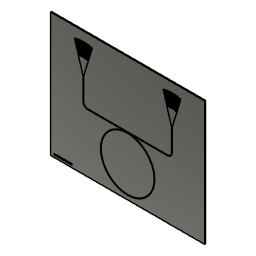
SimpleRes (Autodesk Fusion 360 design; units mm, degrees)
Autodesk Fusion 360 part; units mm, degrees
note: some values were not read from the file. Chosen so that the rebuilt part matches the saved one: which bodies a step acts on.
sketch "Sketch1" plane through (0, 0, 0) normal (0, 1, 0) x (1, 0, 0)
  circle A0 centre (0, 0) radius 30
  circle A1 centre (0, 0) radius 30.5
  line L0 (-45, -30.95) -> (45, -30.95)
  line L1 (-50, -35.95) -> (-50, -60.95)
  line L2 (50, -35.95) -> (50, -60.95)
  arc A2 (-45, -30.95) -> (-50, -35.95) centre (-45, -35.95) ccw
  arc A3 (50, -35.95) -> (45, -30.95) centre (45, -35.95) ccw
  line L3 (49.75, -35.95) -> (49.75, -60.95)
  arc A4 (49.75, -35.95) -> (45, -31.2) centre (45, -35.95) ccw
  line L4 (-45, -31.2) -> (45, -31.2)
  arc A5 (-45, -31.2) -> (-49.75, -35.95) centre (-45, -35.95) ccw
  line L5 (-49.75, -35.95) -> (-49.75, -60.95)
  line L6 (50.25, -35.95) -> (50.25, -60.95)
  arc A6 (50.25, -35.95) -> (45, -30.7) centre (45, -35.95) ccw
  line L7 (-45, -30.7) -> (45, -30.7)
  arc A7 (-45, -30.7) -> (-50.25, -35.95) centre (-45, -35.95) ccw
  line L8 (-50.25, -35.95) -> (-50.25, -60.95)
  line L9 (49.75, -60.95) -> (50.25, -60.95)
  line L10 (50.25, -60.95) -> (60.0334, -92.95)
  line L11 (49.75, -60.95) -> (39.9666, -92.95)
  arc A8 (39.9666, -92.95) -> (60.0334, -92.95) centre (50, -60.95) ccw
  line L12 (-50.25, -60.95) -> (-49.75, -60.95)
  line L13 (-49.75, -60.95) -> (-39.9666, -92.95)
  line L14 (-50.25, -60.95) -> (-60.0334, -92.95)
  arc A9 (-60.0334, -92.95) -> (-39.9666, -92.95) centre (-50, -60.95) ccw
  arc A10 (-55.6371, -78.5703) -> (-44.3629, -78.5703) centre (-50, -60.95) ccw
  arc A11 (-55.698, -78.7608) -> (-44.302, -78.7608) centre (-50, -60.95) ccw
  arc A12 (-55.7589, -78.9512) -> (-44.2411, -78.9512) centre (-50, -60.95) ccw
  arc A13 (-55.8199, -79.1417) -> (-44.1801, -79.1417) centre (-50, -60.95) ccw
  arc A14 (-55.9722, -79.618) -> (-44.0278, -79.618) centre (-50, -60.95) ccw
  arc A15 (-56.0332, -79.8084) -> (-43.9668, -79.8084) centre (-50, -60.95) ccw
  arc A16 (-56.0941, -79.9989) -> (-43.9059, -79.9989) centre (-50, -60.95) ccw
  arc A17 (-56.1551, -80.1894) -> (-43.8449, -80.1894) centre (-50, -60.95) ccw
  arc A18 (-56.3074, -80.6656) -> (-43.6926, -80.6656) centre (-50, -60.95) ccw
  arc A19 (-56.3683, -80.8561) -> (-43.6317, -80.8561) centre (-50, -60.95) ccw
  arc A20 (-56.4293, -81.0466) -> (-43.5707, -81.0466) centre (-50, -60.95) ccw
  arc A21 (-56.4902, -81.2371) -> (-43.5098, -81.2371) centre (-50, -60.95) ccw
  arc A22 (-56.6426, -81.7133) -> (-43.3574, -81.7133) centre (-50, -60.95) ccw
  arc A23 (-56.7035, -81.9038) -> (-43.2965, -81.9038) centre (-50, -60.95) ccw
  arc A24 (-56.7645, -82.0943) -> (-43.2355, -82.0943) centre (-50, -60.95) ccw
  arc A25 (-56.8254, -82.2848) -> (-43.1746, -82.2848) centre (-50, -60.95) ccw
  arc A26 (-56.9778, -82.761) -> (-43.0222, -82.761) centre (-50, -60.95) ccw
  arc A27 (-57.0387, -82.9515) -> (-42.9613, -82.9515) centre (-50, -60.95) ccw
  arc A28 (-57.0996, -83.142) -> (-42.9004, -83.142) centre (-50, -60.95) ccw
  arc A29 (-57.1606, -83.3325) -> (-42.8394, -83.3325) centre (-50, -60.95) ccw
  arc A30 (-57.3129, -83.8087) -> (-42.6871, -83.8087) centre (-50, -60.95) ccw
  arc A31 (-57.3739, -83.9992) -> (-42.6261, -83.9992) centre (-50, -60.95) ccw
  arc A32 (-57.4348, -84.1897) -> (-42.5652, -84.1897) centre (-50, -60.95) ccw
  arc A33 (-57.4958, -84.3802) -> (-42.5042, -84.3802) centre (-50, -60.95) ccw
  arc A34 (-57.6481, -84.8564) -> (-42.3519, -84.8564) centre (-50, -60.95) ccw
  arc A35 (-57.7091, -85.0469) -> (-42.2909, -85.0469) centre (-50, -60.95) ccw
  arc A36 (-57.77, -85.2374) -> (-42.23, -85.2374) centre (-50, -60.95) ccw
  arc A37 (-57.8309, -85.4279) -> (-42.1691, -85.4279) centre (-50, -60.95) ccw
  arc A38 (-57.9833, -85.9041) -> (-42.0167, -85.9041) centre (-50, -60.95) ccw
  arc A39 (-58.0442, -86.0946) -> (-41.9558, -86.0946) centre (-50, -60.95) ccw
  arc A40 (-58.1052, -86.2851) -> (-41.8948, -86.2851) centre (-50, -60.95) ccw
  arc A41 (-58.1661, -86.4756) -> (-41.8339, -86.4756) centre (-50, -60.95) ccw
  arc A42 (-58.3185, -86.9518) -> (-41.6815, -86.9518) centre (-50, -60.95) ccw
  arc A43 (-58.3794, -87.1423) -> (-41.6206, -87.1423) centre (-50, -60.95) ccw
  arc A44 (-58.4403, -87.3328) -> (-41.5597, -87.3328) centre (-50, -60.95) ccw
  arc A45 (-58.5013, -87.5233) -> (-41.4987, -87.5233) centre (-50, -60.95) ccw
  arc A46 (-58.6536, -87.9995) -> (-41.3464, -87.9995) centre (-50, -60.95) ccw
  arc A47 (-58.7146, -88.19) -> (-41.2854, -88.19) centre (-50, -60.95) ccw
  arc A48 (-58.7755, -88.3805) -> (-41.2245, -88.3805) centre (-50, -60.95) ccw
  arc A49 (-58.8365, -88.571) -> (-41.1635, -88.571) centre (-50, -60.95) ccw
  arc A50 (-58.9888, -89.0472) -> (-41.0112, -89.0472) centre (-50, -60.95) ccw
  arc A51 (-59.0498, -89.2377) -> (-40.9502, -89.2377) centre (-50, -60.95) ccw
  arc A52 (-59.1107, -89.4282) -> (-40.8893, -89.4282) centre (-50, -60.95) ccw
  arc A53 (-59.1716, -89.6186) -> (-40.8284, -89.6186) centre (-50, -60.95) ccw
  arc A54 (-59.324, -90.0949) -> (-40.676, -90.0949) centre (-50, -60.95) ccw
  arc A55 (-59.3849, -90.2854) -> (-40.6151, -90.2854) centre (-50, -60.95) ccw
  arc A56 (-59.4459, -90.4758) -> (-40.5541, -90.4758) centre (-50, -60.95) ccw
  arc A57 (-59.5068, -90.6663) -> (-40.4932, -90.6663) centre (-50, -60.95) ccw
  arc A58 (-59.6592, -91.1426) -> (-40.3408, -91.1426) centre (-50, -60.95) ccw
  arc A59 (-59.7201, -91.333) -> (-40.2799, -91.333) centre (-50, -60.95) ccw
  arc A60 (-59.7811, -91.5235) -> (-40.2189, -91.5235) centre (-50, -60.95) ccw
  arc A61 (-59.842, -91.714) -> (-40.158, -91.714) centre (-50, -60.95) ccw
  arc A62 (-59.9943, -92.1902) -> (-40.0057, -92.1902) centre (-50, -60.95) ccw
  arc A63 (-60.0553, -92.3807) -> (-39.9447, -92.3807) centre (-50, -60.95) ccw
  arc A64 (-60.1162, -92.5712) -> (-39.8838, -92.5712) centre (-50, -60.95) ccw
  arc A65 (-60.1772, -92.7617) -> (-39.8228, -92.7617) centre (-50, -60.95) ccw
  arc A66 (44.3629, -78.5703) -> (55.6371, -78.5703) centre (50, -60.95) ccw
  arc A67 (44.302, -78.7608) -> (55.698, -78.7608) centre (50, -60.95) ccw
  arc A68 (44.2411, -78.9512) -> (55.7589, -78.9512) centre (50, -60.95) ccw
  arc A69 (44.1801, -79.1417) -> (55.8199, -79.1417) centre (50, -60.95) ccw
  arc A70 (44.0278, -79.618) -> (55.9722, -79.618) centre (50, -60.95) ccw
  arc A71 (43.9668, -79.8084) -> (56.0332, -79.8084) centre (50, -60.95) ccw
  arc A72 (43.9059, -79.9989) -> (56.0941, -79.9989) centre (50, -60.95) ccw
  arc A73 (43.8449, -80.1894) -> (56.1551, -80.1894) centre (50, -60.95) ccw
  arc A74 (43.6926, -80.6656) -> (56.3074, -80.6656) centre (50, -60.95) ccw
  arc A75 (43.6317, -80.8561) -> (56.3683, -80.8561) centre (50, -60.95) ccw
  arc A76 (43.5707, -81.0466) -> (56.4293, -81.0466) centre (50, -60.95) ccw
  arc A77 (43.5098, -81.2371) -> (56.4902, -81.2371) centre (50, -60.95) ccw
  arc A78 (43.3574, -81.7133) -> (56.6426, -81.7133) centre (50, -60.95) ccw
  arc A79 (43.2965, -81.9038) -> (56.7035, -81.9038) centre (50, -60.95) ccw
  arc A80 (43.2355, -82.0943) -> (56.7645, -82.0943) centre (50, -60.95) ccw
  arc A81 (43.1746, -82.2848) -> (56.8254, -82.2848) centre (50, -60.95) ccw
  arc A82 (43.0222, -82.761) -> (56.9778, -82.761) centre (50, -60.95) ccw
  arc A83 (42.9613, -82.9515) -> (57.0387, -82.9515) centre (50, -60.95) ccw
  arc A84 (42.9004, -83.142) -> (57.0996, -83.142) centre (50, -60.95) ccw
  arc A85 (42.8394, -83.3325) -> (57.1606, -83.3325) centre (50, -60.95) ccw
  arc A86 (42.6871, -83.8087) -> (57.3129, -83.8087) centre (50, -60.95) ccw
  arc A87 (42.6261, -83.9992) -> (57.3739, -83.9992) centre (50, -60.95) ccw
  arc A88 (42.5652, -84.1897) -> (57.4348, -84.1897) centre (50, -60.95) ccw
  arc A89 (42.5042, -84.3802) -> (57.4958, -84.3802) centre (50, -60.95) ccw
  arc A90 (42.3519, -84.8564) -> (57.6481, -84.8564) centre (50, -60.95) ccw
  arc A91 (42.2909, -85.0469) -> (57.7091, -85.0469) centre (50, -60.95) ccw
  arc A92 (42.23, -85.2374) -> (57.77, -85.2374) centre (50, -60.95) ccw
  arc A93 (42.1691, -85.4279) -> (57.8309, -85.4279) centre (50, -60.95) ccw
  arc A94 (42.0167, -85.9041) -> (57.9833, -85.9041) centre (50, -60.95) ccw
  arc A95 (41.9558, -86.0946) -> (58.0442, -86.0946) centre (50, -60.95) ccw
  arc A96 (41.8948, -86.2851) -> (58.1052, -86.2851) centre (50, -60.95) ccw
  arc A97 (41.8339, -86.4756) -> (58.1661, -86.4756) centre (50, -60.95) ccw
  arc A98 (41.6815, -86.9518) -> (58.3185, -86.9518) centre (50, -60.95) ccw
  arc A99 (41.6206, -87.1423) -> (58.3794, -87.1423) centre (50, -60.95) ccw
  arc A100 (41.5597, -87.3328) -> (58.4403, -87.3328) centre (50, -60.95) ccw
  arc A101 (41.4987, -87.5233) -> (58.5013, -87.5233) centre (50, -60.95) ccw
  arc A102 (41.3464, -87.9995) -> (58.6536, -87.9995) centre (50, -60.95) ccw
  arc A103 (41.2854, -88.19) -> (58.7146, -88.19) centre (50, -60.95) ccw
  arc A104 (41.2245, -88.3805) -> (58.7755, -88.3805) centre (50, -60.95) ccw
  arc A105 (41.1635, -88.571) -> (58.8365, -88.571) centre (50, -60.95) ccw
  arc A106 (41.0112, -89.0472) -> (58.9888, -89.0472) centre (50, -60.95) ccw
  arc A107 (40.9502, -89.2377) -> (59.0498, -89.2377) centre (50, -60.95) ccw
  arc A108 (40.8893, -89.4282) -> (59.1107, -89.4282) centre (50, -60.95) ccw
  arc A109 (40.8284, -89.6186) -> (59.1716, -89.6186) centre (50, -60.95) ccw
  arc A110 (40.676, -90.0949) -> (59.324, -90.0949) centre (50, -60.95) ccw
  arc A111 (40.6151, -90.2854) -> (59.3849, -90.2854) centre (50, -60.95) ccw
  arc A112 (40.5541, -90.4758) -> (59.4459, -90.4758) centre (50, -60.95) ccw
  arc A113 (40.4932, -90.6663) -> (59.5068, -90.6663) centre (50, -60.95) ccw
  arc A114 (40.3408, -91.1426) -> (59.6592, -91.1426) centre (50, -60.95) ccw
  arc A115 (40.2799, -91.333) -> (59.7201, -91.333) centre (50, -60.95) ccw
  arc A116 (40.2189, -91.5235) -> (59.7811, -91.5235) centre (50, -60.95) ccw
  arc A117 (40.158, -91.714) -> (59.842, -91.714) centre (50, -60.95) ccw
  arc A118 (40.0057, -92.1902) -> (59.9943, -92.1902) centre (50, -60.95) ccw
  arc A119 (39.9447, -92.3807) -> (60.0553, -92.3807) centre (50, -60.95) ccw
  arc A120 (39.8838, -92.5712) -> (60.1162, -92.5712) centre (50, -60.95) ccw
  arc A121 (39.8228, -92.7617) -> (60.1772, -92.7617) centre (50, -60.95) ccw
  line L15 (-83.2157, 31.3606) -> (-62.7231, 31.3606)
  line L16 (-62.7231, 31.3606) -> (-62.7231, 32.5289)
  line L17 (-62.7231, 32.5289) -> (-83.2157, 32.5289)
  line L18 (-83.2157, 32.5289) -> (-83.2157, 31.3606)
  line L19 (-62.9231, 32.3289) -> (-83.0157, 32.3289)
  line L20 (-83.0157, 32.3289) -> (-83.0157, 31.5606)
  line L21 (-83.0157, 31.5606) -> (-62.9231, 31.5606)
  line L22 (-62.9231, 31.5606) -> (-62.9231, 32.3289)
  line L23 (-73.012, 31.5606) -> (-73.012, 32.3289)
  line L24 (-73.012, 31.5606) -> (-62.9231, 31.5606)
  line L25 (-62.9231, 31.5606) -> (-62.9231, 32.3289)
  line L26 (-62.9231, 32.3289) -> (-73.012, 32.3289)
  line L27 (-73.012, 32.3289) -> (-73.012, 31.5606)
  line L28 (-87.1137, -104.9748) -> (86.8892, -104.9748)
  line L29 (86.8892, -104.9748) -> (86.8892, 35.3192)
  line L30 (86.8892, 35.3192) -> (-87.1137, 35.3192)
  line L31 (-87.1137, 35.3192) -> (-87.1137, -104.9748)
  point P0 (-50, -30.95)
  point P1 (50, -30.95)
  dimension "d1" = 60
  dimension "d2" = 0.5
  dimension "d3" = 30.95
  dimension "d4" = 50
  dimension "d5" = 50
  dimension "d6" = 30
  dimension "d7" = 30
  dimension "d8" = 5
  dimension "d9" = 0.25
  dimension "d10" = -0.25
  dimension "d12" = 107
  dimension "d13" = 107
  dimension "d14" = 32
  dimension "d15" = 32
  dimension "d16" = 107
  dimension "d17" = 107
  dimension "d18" = 32
  dimension "d19" = 32
  dimension "d20" = 18.5
  dimension "d21" = 0.2
  dimension "d22" = 0.4
  dimension "d23" = 0.6
  dimension "d24" = 1.1
  dimension "d25" = 1.3
  dimension "d26" = 1.5
  dimension "d27" = 1.7
  dimension "d28" = 2.2
  dimension "d29" = 2.4
  dimension "d30" = 2.6
  dimension "d31" = 2.8
  dimension "d32" = 3.3
  dimension "d33" = 3.5
  dimension "d34" = 3.7
  dimension "d35" = 3.9
  dimension "d36" = 4.4
  dimension "d37" = 4.6
  dimension "d38" = 4.8
  dimension "d39" = 5
  dimension "d40" = 5.5
  dimension "d41" = 5.7
  dimension "d42" = 5.9
  dimension "d43" = 6.1
  dimension "d44" = 6.6
  dimension "d45" = 6.8
  dimension "d46" = 7
  dimension "d47" = 7.2
  dimension "d48" = 7.7
  dimension "d49" = 7.9
  dimension "d50" = 8.1
  dimension "d51" = 8.3
  dimension "d52" = 8.8
  dimension "d53" = 9
  dimension "d54" = 9.2
  dimension "d55" = 9.4
  dimension "d56" = 9.9
  dimension "d57" = 10.1
  dimension "d58" = 10.3
  dimension "d59" = 10.5
  dimension "d60" = 11
  dimension "d61" = 11.2
  dimension "d62" = 11.4
  dimension "d63" = 11.6
  dimension "d64" = 12.1
  dimension "d65" = 12.3
  dimension "d66" = 12.5
  dimension "d67" = 12.7
  dimension "d68" = 13.2
  dimension "d69" = 13.4
  dimension "d70" = 13.6
  dimension "d71" = 13.8
  dimension "d72" = 14.3
  dimension "d73" = 14.5
  dimension "d74" = 14.7
  dimension "d75" = 14.9
  dimension "d78" = 100
  dimension "d79" = 0
  dimension "d80" = -0.2
  constraint coincident A0.centre A1.centre
  constraint horizontal L0
  constraint perpendicular L0 L1
  constraint perpendicular L0 L2
  constraint coincident P0 L0
  constraint coincident P0 L1
  constraint tangent L0 A2
  constraint tangent L1 A2
  constraint coincident P1 L0
  constraint coincident P1 L2
  constraint tangent L0 A3
  constraint tangent L2 A3
  constraint equal A2 A3
  constraint perpendicular L3 L9
  constraint coincident L2.end A8.centre
  constraint perpendicular L5 L12
  constraint coincident L1.end A9.centre
  constraint coincident L14 A10.start
  constraint coincident L13 A10.end
  constraint horizontal L15
  constraint vertical L16
  constraint horizontal L17
  constraint vertical L18
  constraint coincident L21 L23.start
  constraint coincident L19 L23.end
  constraint perpendicular L19 L23
  constraint horizontal L24
  constraint vertical L25
  constraint horizontal L26
  constraint vertical L27
  constraint horizontal L28
  constraint vertical L29
  constraint horizontal L30
  constraint vertical L31
  measures "d1" diameter of A0
  measures "d3" distance of A0.centre L0
  measures "d4" horizontal distance of A0.centre P1
  measures "d5" horizontal distance of A0.centre P0
  measures "d6" distance of P0 L1.end
  measures "d7" distance of P1 L2.end
  measures "d8" radius of A2
  measures "d12" angle of L9 L10
  measures "d13" angle of L9 L11
  measures "d14" vertical distance of L6.end L10.end
  measures "d15" vertical distance of L2.end L11.end
  measures "d16" angle of L12 L14
  measures "d17" angle of L12 L13
  measures "d18" vertical distance of L5.end L13.end
  measures "d19" vertical distance of L8.end L14.end
  measures "d20" radius of A10
extrude "Extrude1" add sketch "Sketch1" against normal blind 0.22 contours A1 | L0 L1 L2 A2 A3 L6 A6 L7 A7 L8 L9 L12 | L0 L1 L2 A2 A3 L3 A4 L4 A5 L5 L9 L12 | L12 L13 L14 A10 | L9 L10 L11 A66 | L13 L14 A11 A12 | L10 L11 A67 A68 | L13 L14 A13 A14 | L10 L11 A69 A70 | L13 L14 A15 A16 | L10 L11 A71 A72 | L13 L14 A17 A18 | L10 L11 A73 A74 | L13 L14 A19 A20 | L10 L11 A75 A76 | L13 L14 A21 A22 | L10 L11 A77 A78 | L13 L14 A23 A24 | L10 L11 A79 A80 | L13 L14 A25 A26 | L10 L11 A81 A82 | L13 L14 A27 A28 | L10 L11 A83 A84 | L13 L14 A29 A30 | L10 L11 A85 A86 | L13 L14 A31 A32 | L10 L11 A87 A88 | L13 L14 A33 A34 | L10 L11 A89 A90 | L13 L14 A35 A36 | L10 L11 A91 A92 | L13 L14 A37 A38 | L10 L11 A93 A94 | L13 L14 A39 A40 | L10 L11 A95 A96 | L13 L14 A41 A42 | L10 L11 A97 A98 | L13 L14 A43 A44 | L10 L11 A99 A100 | L13 L14 A45 A46 | L10 L11 A101 A102 | L13 L14 A47 A48 | L10 L11 A103 A104 | L13 L14 A49 A50 | L10 L11 A105 A106 | L13 L14 A51 A52 | L10 L11 A107 A108 | L13 L14 A53 A54 | L10 L11 A109 A110 | L13 L14 A55 A56 | L10 L11 A111 A112 | L13 L14 A57 A58 | L10 L11 A113 A114 | L13 L14 A59 A60 | L10 L11 A115 A116 | L13 L14 A61 A62 | L10 L11 A117 A118 | L13 L14 A63 A64 | L10 L11 A119 A120 | L13 L14 A9 A65 | L10 L11 A8 A121 | L15 L16 L17 L18 | L19 L20 L21 L23 L27 makes body 1 at (50.6544, 0, 93.523) makes body 2 at (43.2646, 0, 90.5771) makes body 3 at (56.2613, 0, 88.4323) makes body 4 at (44.2129, 0, 86.2875) makes body 5 at (53.3263, -0.1467, 84.0113) makes body 6 at (47.8373, -0.1467, 81.9389) makes body 7 at (45.749, -0.1467, 79.3657) makes body 8 at (-58.3639, -0.0733, 91.9412) makes body 9 at (-56.6256, -0.1467, 90.1067) makes body 10 at (-56.1507, -0.1467, 87.9585) makes body 11 at (-52.5972, -0.1467, 86.3174) makes body 12 at (-55.2009, -0.1467, 83.6621) makes body 13 at (-52.1627, -0.1467, 81.9389) makes body 14 at (-51.9455, -0.1467, 79.7496) makes body 15 at (-79.8145, 0, -32.0728) makes body 16 at (-45.6353, 0, 79.8529) makes body 17 at (-45.1612, 0, 81.9978) makes body 18 at (-55.313, 0, 84.1426) makes body 19 at (-55.7871, 0, 86.2875) makes body 20 at (-56.2613, 0, 88.4323) makes body 21 at (-56.7354, 0, 90.5771) makes body 22 at (-49.3456, 0, 93.523) makes body 23 at (54.3647, 0, 79.8529) makes body 24 at (45.1612, 0, 81.9978) makes body 25 at (55.313, 0, 84.1426) makes body 26 at (43.0349, -0.0733, 86.6219) makes body 27 at (43.6118, -0.1467, 89.0326) makes body 28 at (46.8597, -0.1467, 91.7905) makes body 29 at (46.6425, -0.1467, 93.9798) makes body 30 at (41.6361, -0.0733, 91.9412) makes body 31 at (43.3744, -0.1467, 90.1067) makes body 32 at (43.8493, -0.1467, 87.9585) makes body 33 at (53.63, -0.1467, 86.1903) makes body 34 at (55.0759, 0, 83.0702) makes body 35 at (45.3982, 0, 80.9254) makes body 36 at (-58.7291, -0.0733, 93.3301) makes body 37 at (-49.3673, 0, 92.425) makes body 38 at (-43.5017, 0, 89.5047) makes body 39 at (-56.0242, 0, 87.3599) makes body 40 at (-55.5501, 0, 85.2151) makes body 41 at (-44.9241, 0, 83.0702) makes body 42 at (-54.6018, 0, 80.9254) makes body 43 at (50.0833, 0, 73.2597) makes body 44 at (-21.122, 0, 21.6654) makes body 45 at (-47.1291, -0.1467, 80.7429) makes body 46 at (-46.8255, -0.1467, 82.9219) makes body 47 at (-52.4886, -0.1467, 85.2228) makes body 48 at (-56.9651, -0.0733, 86.6219) makes body 49 at (-52.923, -0.1467, 89.6013) makes body 50 at (-53.1403, -0.1467, 91.7905) makes body 51 at (-53.3575, -0.1467, 93.9798) makes body 52 at (47.9459, -0.1467, 80.8442) makes body 53 at (53.1745, -0.1467, 82.9219) makes body 54 at (55.5501, 0, 85.2151) makes body 55 at (56.0242, 0, 87.3599) makes body 56 at (56.4983, 0, 89.5047) makes body 57 at (50.6327, 0, 92.425) makes body 58 at (41.2709, -0.0733, 93.3301) makes body 59 at (47.5114, -0.1467, 85.2228)
extrude "Extrude2" add sketch "Sketch1" along normal blind 1 separate body contours A0 | A1 | L0 L1 L2 A2 A3 L6 A6 L7 A7 L8 L9 L12 | L0 L1 L2 A2 A3 L3 A4 L4 A5 L5 L9 L12 | L12 L13 L14 A10 | L9 L10 L11 A66 | L13 L14 A10 A11 | L10 L11 A66 A67 | L13 L14 A11 A12 | L10 L11 A67 A68 | L13 L14 A12 A13 | L10 L11 A68 A69 | L13 L14 A13 A14 | L10 L11 A69 A70 | L13 L14 A14 A15 | L10 L11 A70 A71 | L13 L14 A15 A16 | L10 L11 A71 A72 | L13 L14 A16 A17 | L10 L11 A72 A73 | L13 L14 A17 A18 | L10 L11 A73 A74 | L13 L14 A18 A19 | L10 L11 A74 A75 | L13 L14 A19 A20 | L10 L11 A75 A76 | L13 L14 A20 A21 | L10 L11 A76 A77 | L13 L14 A21 A22 | L10 L11 A77 A78 | L13 L14 A22 A23 | L10 L11 A78 A79 | L13 L14 A23 A24 | L10 L11 A79 A80 | L13 L14 A24 A25 | L10 L11 A80 A81 | L13 L14 A25 A26 | L10 L11 A81 A82 | L13 L14 A26 A27 | L10 L11 A82 A83 | L13 L14 A27 A28 | L10 L11 A83 A84 | L13 L14 A28 A29 | L10 L11 A84 A85 | L13 L14 A29 A30 | L10 L11 A85 A86 | L13 L14 A30 A31 | L10 L11 A86 A87 | L13 L14 A31 A32 | L10 L11 A87 A88 | L13 L14 A32 A33 | L10 L11 A88 A89 | L13 L14 A33 A34 | L10 L11 A89 A90 | L13 L14 A34 A35 | L10 L11 A90 A91 | L13 L14 A35 A36 | L10 L11 A91 A92 | L13 L14 A36 A37 | L10 L11 A92 A93 | L13 L14 A37 A38 | L10 L11 A93 A94 | L13 L14 A38 A39 | L10 L11 A94 A95 | L13 L14 A39 A40 | L10 L11 A95 A96 | L13 L14 A40 A41 | L10 L11 A96 A97 | L13 L14 A41 A42 | L10 L11 A97 A98 | L13 L14 A42 A43 | L10 L11 A98 A99 | L13 L14 A43 A44 | L10 L11 A99 A100 | L13 L14 A44 A45 | L10 L11 A100 A101 | L13 L14 A45 A46 | L10 L11 A101 A102 | L13 L14 A46 A47 | L10 L11 A102 A103 | L13 L14 A47 A48 | L10 L11 A103 A104 | L13 L14 A48 A49 | L10 L11 A104 A105 | L13 L14 A49 A50 | L10 L11 A105 A106 | L13 L14 A50 A51 | L10 L11 A106 A107 | L13 L14 A51 A52 | L10 L11 A107 A108 | L13 L14 A52 A53 | L10 L11 A108 A109 | L13 L14 A53 A54 | L10 L11 A109 A110 | L13 L14 A54 A55 | L10 L11 A110 A111 | L13 L14 A55 A56 | L10 L11 A111 A112 | L13 L14 A56 A57 | L10 L11 A112 A113 | L13 L14 A57 A58 | L10 L11 A113 A114 | L13 L14 A58 A59 | L10 L11 A114 A115 | L13 L14 A59 A60 | L10 L11 A115 A116 | L13 L14 A60 A61 | L10 L11 A116 A117 | L13 L14 A61 A62 | L10 L11 A117 A118 | L13 L14 A62 A63 | L10 L11 A118 A119 | L13 L14 A63 A64 | L10 L11 A119 A120 | L13 L14 A64 A65 | L10 L11 A120 A121 | L13 L14 A9 A65 | L10 L11 A8 A121 | L15 L16 L17 L18 | L19 L21 L22 L23 L24 L25 L26 L27 | L19 L20 L21 L23 L27 | L28 L29 L30 L31 makes body 60
combine "Combine1" operation add target body 1 tool bodies 48 30 53 49 39 36 3 43 46 10 13 45 31 12 makes body 61 at (-52.1627, -0.1467, 81.9389) makes body 62 at (-46.8255, -0.1467, 82.9219) makes body 63 at (56.2613, 0, 88.4323) makes body 64 at (-56.0242, 0, 87.3599) makes body 65 at (53.1745, -0.1467, 82.9219) makes body 66 at (-56.9651, -0.0733, 86.6219) makes body 67 at (43.3744, -0.1467, 90.1067) makes body 68 at (41.6361, -0.0733, 91.9412) makes body 69 at (-52.923, -0.1467, 89.6013) makes body 70 at (-58.7291, -0.0733, 93.3301) makes body 71 at (50.0833, 0, 73.2597) makes body 72 at (-56.1507, -0.1467, 87.9585) makes body 73 at (-47.1291, -0.1467, 80.7429) makes body 74 at (-55.2009, -0.1467, 83.6621)
combine "Combine2" operation add target body 8 tool bodies 29 38 58 25 56 33 55 37 23 28 34 24 19 27 59 9 4 20 54 32 14 17 44 26 2 41 50 7 16 21 42 22 5 40 18 52 35 6 57 47 51 11 makes body 75 at (50.6327, 0, 92.425) makes body 76 at (45.3982, 0, 80.9254) makes body 77 at (-55.313, 0, 84.1426) makes body 78 at (53.3263, -0.1467, 84.0113) makes body 79 at (-54.6018, 0, 80.9254) makes body 80 at (-45.6353, 0, 79.8529) makes body 81 at (-53.1403, -0.1467, 91.7905) makes body 82 at (43.2646, 0, 90.5771) makes body 83 at (-21.122, 0, 21.6654) makes body 84 at (-51.9455, -0.1467, 79.7496) makes body 85 at (55.5501, 0, 85.2151) makes body 86 at (44.2129, 0, 86.2875) makes body 87 at (47.5114, -0.1467, 85.2228) makes body 88 at (-55.7871, 0, 86.2875) makes body 89 at (55.0759, 0, 83.0702) makes body 90 at (54.3647, 0, 79.8529) makes body 91 at (56.0242, 0, 87.3599) makes body 92 at (56.4983, 0, 89.5047) makes body 93 at (41.2709, -0.0733, 93.3301) makes body 94 at (46.6425, -0.1467, 93.9798) makes body 95 at (-53.3575, -0.1467, 93.9798) makes body 96 at (-43.5017, 0, 89.5047) makes body 97 at (55.313, 0, 84.1426) makes body 98 at (53.63, -0.1467, 86.1903) makes body 99 at (-49.3673, 0, 92.425) makes body 100 at (46.8597, -0.1467, 91.7905) makes body 101 at (45.1612, 0, 81.9978) makes body 102 at (43.6118, -0.1467, 89.0326) makes body 103 at (-56.6256, -0.1467, 90.1067) makes body 104 at (-56.2613, 0, 88.4323) makes body 105 at (43.8493, -0.1467, 87.9585) makes body 106 at (-45.1612, 0, 81.9978) makes body 107 at (43.0349, -0.0733, 86.6219) makes body 108 at (-44.9241, 0, 83.0702) makes body 109 at (45.749, -0.1467, 79.3657) makes body 110 at (-56.7354, 0, 90.5771) makes body 111 at (-49.3456, 0, 93.523) makes body 112 at (-55.5501, 0, 85.2151) makes body 113 at (47.9459, -0.1467, 80.8442) makes body 114 at (47.8373, -0.1467, 81.9389) makes body 115 at (-52.4886, -0.1467, 85.2228) makes body 116 at (-52.5972, -0.1467, 86.3174)
combine "Combine3" operation add target body 61 tool bodies 77 106 89 83 95 87 92 97 105 112 114 103 78 91 82 84 81 85 94 96 98 104 88 79 86 99 102 107 93 108 75 80 101 76 90 100 109 110 111 113 115 116 64 62 63 70 74 69 71 68 73 67 66 72 65 makes body 117 at (43.3744, -0.1467, 90.1067) makes body 118 at (41.6361, -0.0733, 91.9412) makes body 119 at (-52.923, -0.1467, 89.6013) makes body 120 at (-58.7291, -0.0733, 93.3301) makes body 121 at (-46.8255, -0.1467, 82.9219) makes body 122 at (-52.5972, -0.1467, 86.3174) makes body 123 at (47.9459, -0.1467, 80.8442) makes body 124 at (-56.7354, 0, 90.5771) makes body 125 at (46.8597, -0.1467, 91.7905) makes body 126 at (45.3982, 0, 80.9254) makes body 127 at (-45.6353, 0, 79.8529) makes body 128 at (-44.9241, 0, 83.0702) makes body 129 at (43.0349, -0.0733, 86.6219) makes body 130 at (-49.3673, 0, 92.425) makes body 131 at (-54.6018, 0, 80.9254) makes body 132 at (-56.2613, 0, 88.4323) makes body 133 at (-43.5017, 0, 89.5047) makes body 134 at (55.5501, 0, 85.2151) makes body 135 at (-51.9455, -0.1467, 79.7496) makes body 136 at (56.0242, 0, 87.3599) makes body 137 at (-56.6256, -0.1467, 90.1067) makes body 138 at (-55.5501, 0, 85.2151) makes body 139 at (55.313, 0, 84.1426) makes body 140 at (47.5114, -0.1467, 85.2228) makes body 141 at (-21.122, 0, 21.6654) makes body 142 at (-45.1612, 0, 81.9978) makes body 143 at (-56.1507, -0.1467, 87.9585) makes body 144 at (-55.313, 0, 84.1426) makes body 145 at (55.0759, 0, 83.0702) makes body 146 at (-53.3575, -0.1467, 93.9798) makes body 147 at (56.4983, 0, 89.5047) makes body 148 at (43.8493, -0.1467, 87.9585) makes body 149 at (47.8373, -0.1467, 81.9389) makes body 150 at (53.3263, -0.1467, 84.0113) makes body 151 at (43.2646, 0, 90.5771) makes body 152 at (-53.1403, -0.1467, 91.7905) makes body 153 at (46.6425, -0.1467, 93.9798) makes body 154 at (53.63, -0.1467, 86.1903) makes body 155 at (-55.7871, 0, 86.2875) makes body 156 at (44.2129, 0, 86.2875) makes body 157 at (43.6118, -0.1467, 89.0326) makes body 158 at (41.2709, -0.0733, 93.3301) makes body 159 at (50.6327, 0, 92.425) makes body 160 at (45.1612, 0, 81.9978) makes body 161 at (54.3647, 0, 79.8529) makes body 162 at (45.749, -0.1467, 79.3657) makes body 163 at (-49.3456, 0, 93.523) makes body 164 at (-52.4886, -0.1467, 85.2228) makes body 165 at (-56.0242, 0, 87.3599) makes body 166 at (56.2613, 0, 88.4323) makes body 167 at (-55.2009, -0.1467, 83.6621) makes body 168 at (50.0833, 0, 73.2597) makes body 169 at (-47.1291, -0.1467, 80.7429) makes body 170 at (-56.9651, -0.0733, 86.6219) makes body 171 at (53.1745, -0.1467, 82.9219)
combine "Combine4" operation add target body 8 tool bodies 1 makes body 172 at (50.6544, 0, 93.523)
sketch "Sketch2" plane through (0, 0, 0) normal (0, -1, 0) x (1, 0, 0)
  line L0 (-87.1137, 104.9748) -> (-87.1137, -35.3192)
  line L1 (-87.1137, -35.3192) -> (86.8892, -35.3192)
  line L2 (86.8892, -35.3192) -> (86.8892, 104.9748)
  line L3 (86.8892, 104.9748) -> (-87.1137, 104.9748)
  line L4 (-69.5, -30.5) -> (-62.7446, -30.5)
  line L5 (-69.1517, -30.5) -> (-62.7712, -30.5) construction
  line L6 (-62.7712, -30.5) -> (-62.7712, -28.788) construction
  line L7 (-62.7712, -28.788) -> (-69.1517, -28.788) construction
  line L8 (-69.1517, -28.788) -> (-69.1517, -30.5) construction
  dimension "d85" = 1.6
  text T0 "20 μm" font "Arial" height 1.6 align left top in box 6.3805 x 1.712 at (-69.1517, -30.5) x (1, 0) y (0, 1) spacing 1
  constraint horizontal L4
  constraint coincident L4
extrude "Extrude3" add sketch "Sketch2" along normal blind 0.22 separate body text T0 makes body 173 at (-67.7443, 0, -29.7391) makes body 174 at (-65.8716, 0, -29.9852) makes body 175 at (-64.6113, 0, -29.8012) makes body 176 at (-68.708, 0, -30.3251)
equation "d3 = 30 mm + 0.5 mm + 0.2 mm + 0.25 mm"
equation "d24 = 0.6 mm + 0.5 mm"
named bodies: "Escala", "Base"
